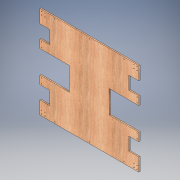
# Autodesk Inventor part: Belly Pan V2
Saved by Autodesk Inventor 2018 (Build 220112000, 112)
## iProperties
Created: 2018-12-20
Part Number: Belly Pan V2
Material: Generic
Document SubType Name: Modeling
Designer: maste
Density: 1 g/cm^3
Appearance: Default
Author: maste
Autodesk Inventor part; units mm, degrees
ref_plane "YZ Plane" through (0, 0, 0) normal (1, 0, 0) x (0, 1, 0)
ref_plane "XZ Plane" through (0, 0, 0) normal (0, 1, 0) x (-1, 0, 0)
ref_plane "XY Plane" through (0, 0, 0) normal (0, 0, 1) x (1, 0, 0)
sketch "Sketch1" plane through (0, 0, 0) normal (0, 0, 1) x (1, 0, 0)
  line L0 (0, 0) -> (762, 0)
  line L1 (0, 0) -> (0, -101.6)
  line L2 (0, -101.6) -> (76.2, -101.6)
  line L3 (76.2, -101.6) -> (76.2, -203.2)
  line L4 (76.2, -203.2) -> (0, -203.2)
  line L5 (0, -203.2) -> (0, -266.7)
  line L6 (0, -266.7) -> (228.6, -266.7)
  line L7 (228.6, -266.7) -> (228.6, -355.6)
  line L8 (0, -711.2) -> (762, -711.2)
  line L9 (0, -711.2) -> (0, -609.6)
  line L10 (0, -609.6) -> (76.2, -609.6)
  line L11 (76.2, -609.6) -> (76.2, -508)
  line L12 (76.2, -508) -> (0, -508)
  line L13 (0, -508) -> (0, -444.5)
  line L14 (0, -444.5) -> (228.6, -444.5)
  line L15 (228.6, -444.5) -> (228.6, -355.6)
  line L16 (762, 0) -> (762, -101.6)
  line L17 (762, -101.6) -> (685.8, -101.6)
  line L18 (685.8, -101.6) -> (685.8, -203.2)
  line L19 (685.8, -203.2) -> (762, -203.2)
  line L20 (762, -203.2) -> (762, -266.7)
  line L21 (762, -266.7) -> (533.4, -266.7)
  line L22 (533.4, -266.7) -> (533.4, -355.6)
  line L23 (762, -711.2) -> (762, -609.6)
  line L24 (762, -609.6) -> (685.8, -609.6)
  line L25 (685.8, -609.6) -> (685.8, -508)
  line L26 (685.8, -508) -> (762, -508)
  line L27 (762, -508) -> (762, -444.5)
  line L28 (762, -444.5) -> (533.4, -444.5)
  line L29 (533.4, -444.5) -> (533.4, -355.6)
  dimension "d0" = 762
  dimension "d1" = 101.6
  dimension "d2" = 76.2
  dimension "d3" = 101.6
  dimension "d4" = 63.5
  dimension "d5" = 228.6
  dimension "d7" = 88.9
  constraints: 60 end point, 8 point on line, 4 perpendicular, 2 vertical, 1 horizontal
  measures "d0" distance of L0.start L0.end
  measures "d1" distance of L0.start L1.end
  measures "d2" distance of L1.end L2.end
  measures "d3" distance of L2.end L3.end
  measures "d4" distance of L4.end L5.end
  measures "d5" distance of L5.end L6.end
  measures "d7" distance of L6.end L7.end
extrude "Extrusion1" add sketch "Sketch1" along normal blind 9.525
sketch "Sketch2" plane through (0, 0, 9.525) normal (0, 0, 1) x (1, 0, 0)
  line L0 (0, 0) -> (12.7, 0)
  line L1 (0, 0) -> (762, 0) projected
  line L2 (12.7, 0) -> (12.7, -12.7)
  line L3 (12.7, -12.7) -> (38.1, -12.7)
  line L4 (38.1, -12.7) -> (38.1, -38.1)
  line L5 (38.1, -38.1) -> (12.7, -38.1)
  circle A0 centre (12.7, -12.7) radius 2.54
  circle A1 centre (38.1, -12.7) radius 2.54
  circle A2 centre (38.1, -38.1) radius 2.54
  circle A3 centre (12.7, -38.1) radius 2.54
  line L6 (0, -203.2) -> (76.2, -203.2) projected
  line L7 (0, -203.2) -> (12.7, -203.2)
  line L8 (12.7, -203.2) -> (12.7, -215.9)
  line L9 (228.6, -266.7) -> (0, -266.7) projected
  line L10 (0, -266.7) -> (12.7, -266.7)
  line L11 (12.7, -266.7) -> (12.7, -254)
  circle A4 centre (12.7, -254) radius 2.54
  circle A5 centre (12.7, -215.9) radius 2.54
  line L12 (381, 0) -> (381, -711.2)
  line L13 (762, -711.2) -> (0, -711.2) projected
  line L14 (0, -355.6) -> (762, -355.6)
  line L15 (762, 0) -> (749.3, 0)
  line L16 (762, 0) -> (0, 0)
  line L17 (749.3, 0) -> (749.3, -12.7)
  line L18 (749.3, -12.7) -> (723.9, -12.7)
  line L19 (723.9, -12.7) -> (723.9, -38.1)
  line L20 (723.9, -38.1) -> (749.3, -38.1)
  circle A6 centre (749.3, -12.7) radius 2.54
  circle A7 centre (723.9, -12.7) radius 2.54
  circle A8 centre (723.9, -38.1) radius 2.54
  circle A9 centre (749.3, -38.1) radius 2.54
  line L21 (762, -203.2) -> (685.8, -203.2)
  line L22 (762, -203.2) -> (749.3, -203.2)
  line L23 (749.3, -203.2) -> (749.3, -215.9)
  line L24 (533.4, -266.7) -> (762, -266.7)
  line L25 (762, -266.7) -> (749.3, -266.7)
  line L26 (749.3, -266.7) -> (749.3, -254)
  circle A10 centre (749.3, -254) radius 2.54
  circle A11 centre (749.3, -215.9) radius 2.54
  line L27 (0, -711.2) -> (12.7, -711.2)
  line L28 (0, -711.2) -> (762, -711.2)
  line L29 (12.7, -711.2) -> (12.7, -698.5)
  line L30 (12.7, -698.5) -> (38.1, -698.5)
  line L31 (38.1, -698.5) -> (38.1, -673.1)
  line L32 (38.1, -673.1) -> (12.7, -673.1)
  circle A12 centre (12.7, -698.5) radius 2.54
  circle A13 centre (38.1, -698.5) radius 2.54
  circle A14 centre (38.1, -673.1) radius 2.54
  circle A15 centre (12.7, -673.1) radius 2.54
  line L33 (0, -508) -> (76.2, -508)
  line L34 (0, -508) -> (12.7, -508)
  line L35 (12.7, -508) -> (12.7, -495.3)
  line L36 (228.6, -444.5) -> (0, -444.5)
  line L37 (0, -444.5) -> (12.7, -444.5)
  line L38 (12.7, -444.5) -> (12.7, -457.2)
  circle A16 centre (12.7, -457.2) radius 2.54
  circle A17 centre (12.7, -495.3) radius 2.54
  line L39 (381, -711.2) -> (381, 0)
  line L40 (762, -711.2) -> (749.3, -711.2)
  line L41 (762, -711.2) -> (0, -711.2)
  line L42 (749.3, -711.2) -> (749.3, -698.5)
  line L43 (749.3, -698.5) -> (723.9, -698.5)
  line L44 (723.9, -698.5) -> (723.9, -673.1)
  line L45 (723.9, -673.1) -> (749.3, -673.1)
  circle A18 centre (749.3, -698.5) radius 2.54
  line L46 (533.4, -444.5) -> (762, -444.5)
  line L47 (749.3, -444.5) -> (749.3, -457.2)
  line L48 (762, -444.5) -> (749.3, -444.5)
  circle A19 centre (749.3, -457.2) radius 2.54
  circle A20 centre (749.3, -495.3) radius 2.54
  line L49 (749.3, -508) -> (749.3, -495.3)
  line L50 (762, -508) -> (685.8, -508)
  line L51 (762, -508) -> (749.3, -508)
  circle A21 centre (723.9, -673.1) radius 2.54
  circle A22 centre (723.9, -698.5) radius 2.54
  circle A23 centre (749.3, -673.1) radius 2.54
  dimension "d10" = 12.7
  dimension "d11" = 12.7
  dimension "d12" = 25.4
  dimension "d13" = 25.4
  dimension "d14" = 25.4
  dimension "d16" = 5.08
  dimension "d17" = 12.7
  dimension "d18" = 12.7
  dimension "d19" = 12.7
  constraints: 96 end point, 65 symmetric about line, 24 centre point, 24 coincident, 16 point on line, 5 perpendicular, 2 midpoint, 1 horizontal, 18 other
  measures "d10" distance of L0.start L0.end
  measures "d11" distance of L0.end L2.end
  measures "d12" distance of L2.end L3.end
  measures "d13" distance of L3.end L4.end
  measures "d14" distance of L4.end L5.end
  measures "d16" diameter of A0
  measures "d17" distance of L6.start L7.end
  measures "d18" distance of L7.end L8.end
  measures "d19" distance of L10.end L11.end
extrude "Extrusion2" cut sketch "Sketch2" against normal blind 9.525
sketch "Sketch3" plane through (0, 0, 9.525) normal (0, 0, 1) x (1, 0, 0)
  line L0 (0, 0) -> (762, 0) projected
  line L1 (0, 0) -> (0, -12.7)
  line L2 (0, -101.6) -> (0, 0) projected
  line L3 (0, -12.7) -> (114.3, -12.7)
  line L4 (114.3, -12.7) -> (381, -12.7)
  line L5 (381, -12.7) -> (647.7, -12.7)
  line L6 (0, 0) -> (0, -355.6)
  line L7 (0, -355.6) -> (797.2248, -355.6)
  circle A0 centre (114.3, -12.7) radius 2.54
  circle A1 centre (381, -12.7) radius 2.54
  circle A2 centre (647.7, -12.7) radius 2.54
  circle A3 centre (114.3, -698.5) radius 2.54
  circle A4 centre (381, -698.5) radius 2.54
  circle A5 centre (647.7, -698.5) radius 2.54
  dimension "d22" = 12.7
  dimension "d23" = 114.3
  dimension "d24" = 266.7
  dimension "d25" = 355.6
  dimension "d28" = 5.08
  constraints: 12 end point, 6 centre point, 3 coincident, 3 point on line, 3 symmetric about line, 2 perpendicular, 1 vertical, 3 other
  measures "d22" distance of L0.start L1.end
  measures "d23" distance of L1.end L3.end
  measures "d24" distance of L4.end L5.end
  measures "d25" distance of L0.start L6.end
  measures "d28" diameter of A0
extrude "Extrusion3" cut sketch "Sketch3" against normal blind 9.525
body "Solid1"
